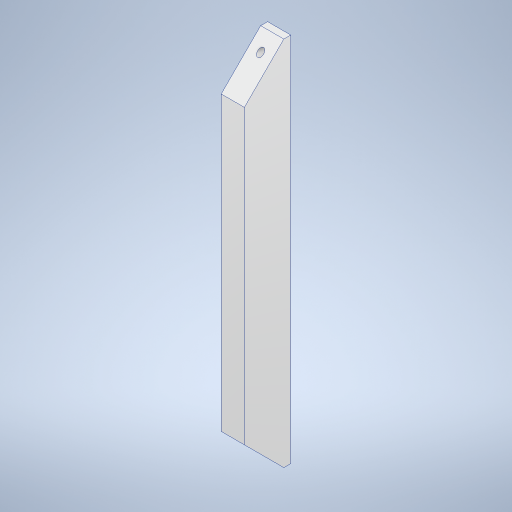
# Autodesk Inventor part: slanted_alum_bar
Saved by Autodesk Inventor 2024 (Build 280153000, 153)
## iProperties
Created: 2023-11-20
Part Number: slanted_alum_bar
Material: Generic
Document SubType Name: Modeling
Designer: s137416
Density: 1 g/cm^3
Appearance: Aluminum - Flat
Author: s137416
Autodesk Inventor part; units mm, degrees
ref_plane "YZ Plane" through (0, 0, 0) normal (1, 0, 0) x (0, 1, 0)
ref_plane "XZ Plane" through (0, 0, 0) normal (0, 1, 0) x (-1, 0, 0)
ref_plane "XY Plane" through (0, 0, 0) normal (0, 0, 1) x (1, 0, 0)
sketch "Sketch1" plane through (0, 0, 0) normal (0, 1, 0) x (-1, 0, 0)
  line L0 (7.1515, 37.8857) -> (-18.2485, 37.8857)
  line L1 (-18.2485, 37.8857) -> (-18.2485, -12.9143)
  line L2 (-18.2485, -12.9143) -> (7.1515, -12.9143)
  line L3 (7.1515, -12.9143) -> (7.1515, 37.8857)
  point P0 (0, 0)
  dimension "d0" = 25.4
  dimension "d1" = 50.8
  constraints: 8 end point, 2 parallel, 1 horizontal, 1 perpendicular
  measures "d0" distance of L2.end L1.end
  measures "d1" distance of L2.end L0.start
extrude "Extrusion1" add sketch "Sketch1" along normal blind 406.4
chamfer "Chamfer1" distance 43.18 angle 45 2 edges at (5.5485, 406.4, 37.8857) (5.5485, 0, 37.8857)
sketch "Sketch2" plane through (-7.1515, 43.18, 37.8857) normal (0, 0, 1) x (1, 0, 0)
  circle A0 centre (12.7, 350.52) radius 3.175
  line L0 (25.4, 363.22) -> (0, 363.22) projected
  circle A1 centre (12.7, -30.48) radius 3.175
  line L1 (0, -43.18) -> (25.4, -43.18) projected
  point P0 (7.1515, -43.18)
  dimension "d7" = 6.35
  dimension "d8" = 12.7
  dimension "d9" = 6.35
  dimension "d10" = 12.7
  constraints: 2 centre point
  measures "d7" diameter of A0
  measures "d8" distance from line of L0 A0.centre
  measures "d9" diameter of A1
  measures "d10" distance from line of L1 A1.centre
hole "Hole1" at (5.5485, 393.7, 37.8857) at (5.5485, 12.7, 37.8857) direction (0, 0, -1) diameter 6.35 end through all
body "Solid1"
